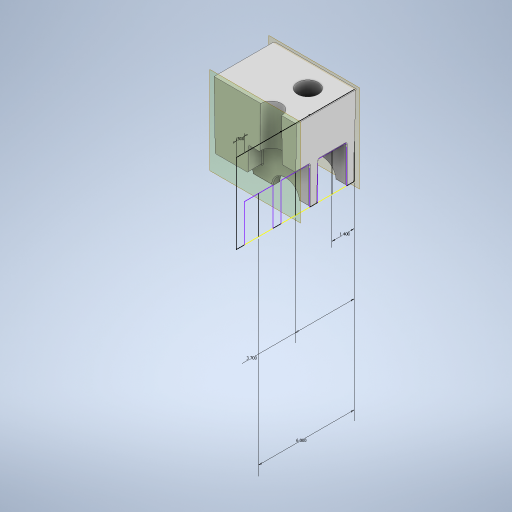
# Autodesk Inventor part: E.Engine Block Top Cast Image Left
Saved by Autodesk Inventor 2023 (Build 270158000, 158)
## iProperties
Created: 2023-01-04
Part Number: E.Engine Block Top Cast Image Left
Material: Generic
Document SubType Name: Modeling
Designer: tgr41
Density: 1 g/cm^3
Appearance: Default
Mass: 2134.37 g
Surface Area: 1668.76 cm^2
Volume: 2134.37 cm^3
Author: tgr41
Autodesk Inventor part; units mm, degrees
ref_plane "YZ Plane" through (0, 0, 0) normal (1, 0, 0) x (0, 1, 0)
ref_plane "XZ Plane" through (0, 0, 0) normal (0, 1, 0) x (-1, 0, 0)
sketch "Sketch1" plane through (0, 0, 0) normal (0, 0, 1) x (1, 0, 0)
  line L0 (127, 0) -> (127, 127)
  line L1 (127, 127) -> (0, 127)
  line L2 (0, 127) -> (0, 0)
  arc A0 (109.5375, 0) -> (68.2625, 0) centre (88.9, 0) ccw
  arc A1 (36.3964, 0) -> (14.4, 0) centre (25.3982, 0) ccw
  line L3 (14.4, 0) -> (0, 0)
  line L4 (127, 0) -> (109.5375, 0)
  line L5 (68.2625, 0) -> (36.3964, 0)
  dimension "d0" = 127
  dimension "d2" = 41.275
  dimension "d25" = 38.1
  dimension "d26" = 21.9964
  dimension "d30" = 127
  constraints: 12 end point, 4 point on circle, 3 horizontal, 2 centre point, 1 parallel
  measures "d0" distance of L1.end L0.end
  measures "d2" diameter of A0
  measures "d25" distance from line of L0 A0.centre
  measures "d26" diameter of A1
  measures "d30" distance between parallel lines of L1 L3
extrude "Extrusion1" add sketch "Sketch1" along normal blind 187.96
sketch "Sketch2" plane through (0, 127, 0) normal (0, 1, 0) x (1, 0, 0)
  circle A0 centre (88.9, -152.4) radius 17.78
  line L0 (127, -187.96) -> (0, -187.96) projected
  line L1 (127, 0) -> (127, -187.96) projected
  circle A1 centre (88.9, -93.98) radius 17.78
  circle A2 centre (88.9, -35.56) radius 17.78
  line L2 (127, 0) -> (0, 0) projected
  point P0 (127, -35.56)
  point P1 (127, -93.98)
  point P2 (127, -152.4)
  dimension "d6" = 35.56
  dimension "d7" = 38.1
  dimension "d10" = 35.56
  dimension "d11" = 38.1
  dimension "d13" = 58.42
  dimension "d14" = 38.1
  dimension "d29" = 35.56
  constraints: 3 centre point, 2 equal radius, 2 point on line, 1 midpoint
  measures "d6" distance from line of L0 A0.centre
  measures "d7" distance from line of L1 A0.centre
  measures "d10" distance from line of L2 A2.centre
  measures "d11" distance from line of L1 A2.centre
  measures "d13" distance of A1.centre A0.centre
  measures "d14" distance from line of L1 A1.centre
  measures "d29" diameter of A2
sketch "Sketch3" plane through (127, 0, 0) normal (1, 0, 0) x (0, 0, -1)
  line L0 (0, 127) -> (-187.96, 127) projected
  line L1 (0, 0) -> (-187.96, 0) projected
  line L2 (-35.56, 59.69) -> (-35.56, 0)
  line L3 (0, 0) -> (-187.96, 0) projected
  line L4 (-93.98, 0) -> (-93.98, 59.69)
  line L5 (-152.4, 59.69) -> (-152.4, 0)
  line L6 (0, 0) -> (0, 127) projected
  line L7 (-187.96, 0) -> (-175.26, 0)
  line L8 (-175.26, 0) -> (-175.26, 59.69)
  line L9 (-175.26, 127) -> (-187.96, 127)
  line L10 (-187.96, 127) -> (-187.96, 0)
  line L11 (-116.84, 0) -> (-129.54, 0)
  line L12 (-129.54, 0) -> (-129.54, 59.69)
  line L13 (-129.54, 127) -> (-116.84, 127)
  line L14 (-116.84, 59.69) -> (-116.84, 0)
  line L15 (-35.56, 59.69) -> (-35.56, 0)
  line L16 (0, 0) -> (-12.7, 0)
  line L17 (-12.7, 0) -> (-12.7, 59.69)
  line L18 (-12.7, 127) -> (0, 127)
  line L19 (0, 127) -> (0, 0)
  line L20 (-71.12, 0) -> (-58.42, 0)
  line L21 (-58.42, 0) -> (-58.42, 59.69)
  line L22 (-58.42, 127) -> (-71.12, 127)
  line L23 (-71.12, 59.69) -> (-71.12, 0)
  line L24 (-187.96, 127) -> (-187.96, 0) projected
  line L25 (-187.96, 127) -> (0, 127)
  line L26 (-58.42, 59.69) -> (-12.7, 59.69)
  line L27 (-175.26, 59.69) -> (-129.54, 59.69)
  line L28 (-116.84, 59.69) -> (-71.12, 59.69)
  dimension "d15" = 35.56
  dimension "d16" = 93.98
  dimension "d17" = 152.4
  dimension "d18" = 12.7
  constraints: 48 end point, 14 symmetric about line, 7 perpendicular, 4 midpoint, 3 point on line, 2 horizontal, 2 parallel
  measures "d15" distance between parallel lines of L6 L2
  measures "d16" distance between parallel lines of L6 L4
  measures "d17" distance between parallel lines of L6 L5
  measures "d18" distance of L9.end L9.start
extrude "Extrusion2" cut sketch "Sketch3" against normal blind 187.96 contours L1 L2 L26 L17 | L1 L21 L26 L2 | L1 L4 L28 L23 | L1 L14 L28 L4 | L1 L5 L27 L12 | L8 L27 L5 L1
extrude "Extrusion3" cut sketch "Sketch2" against normal blind 187.96
sketch "Sketch4" plane through (127, 59.69, 129.54) normal (0, -1, 0) x (1, 0, 0)
  line L0 (-58.7375, -116.84) -> (-90.6036, -116.84) projected
  line L1 (-74.6705, -116.84) -> (-74.6705, 45.72)
  line L2 (-90.6036, 45.72) -> (-58.7375, 45.72) projected
  line L3 (-74.6705, 45.72) -> (-127, 45.72)
  line L4 (-127, -116.84) -> (-127, -71.12) projected
  line L5 (-127, 45.72) -> (-127, -116.84)
  line L6 (-127, -116.84) -> (-74.6705, -116.84)
  point P0 (-127, -129.54)
  point P1 (-127, -71.12)
  constraints: 8 end point, 2 midpoint, 1 collinear, 1 horizontal, 1 perpendicular
extrude "Extrusion4" add sketch "Sketch4" along normal blind 38.1
draft "FaceDraft1" angle -1 pull direction (0, 1, 0) faces at (69.5273, 91.0988, 187.96) (0, 91.8633, 86.36) (127, 104.5633, 86.36) (69.5273, 91.0988, 0) (106.6223, 82.1267, 36.9907) (106.6223, 82.1267, 95.4107) (106.6223, 82.1267, 153.8307) fixed edges at (52.3295, 0, 187.96) (0, 0, 64.77) (127, 0, 6.35) (52.3295, 0, 0) (71.12, 59.69, 35.56) (71.12, 59.69, 93.98) (71.12, 59.69, 152.4)
draft "FaceDraft2" angle 1 pull direction (0, -1, 0) faces at (90.5863, 46.6223, 116.84) (90.5863, 46.6223, 129.54) fixed edges at (52.3295, 0, 116.84) (52.3295, 0, 129.54)
draft "FaceDraft3" angle 1 pull direction (0, -1, 0) faces at (90.5863, 46.6223, 58.42) (90.5863, 46.6223, 71.12) fixed edges at (118.2687, 0, 58.42) (118.2687, 0, 71.12)
draft "FaceDraft4" angle 1 pull direction (0, -1, 0) faces at (90.5863, 46.6223, 12.7) fixed edges at (52.3295, 0, 12.7)
draft "FaceDraft5" angle 1 pull direction (0, -1, 0) faces at (90.5863, 46.6223, 175.26) fixed edges at (52.3295, 0, 175.26)
draft "FaceDraft6" angle 1 pull direction (0, -1, 0) faces at (52.3295, 34.29, 42.8327) (52.3295, 34.29, 101.2527) (52.3295, 34.29, 159.6727) fixed edges at (52.3295, 21.59, 35.56) (52.3295, 21.59, 93.98) (52.3295, 21.59, 152.4)
fillet "Fillet1" radius 1.5875 89 edges at (52.9945, 59.69, 152.4) (52.662, 40.64, 130.2494) (90.5182, 59.69, 130.5819) (52.9945, 59.69, 93.98) (52.662, 40.64, 71.8294) (90.5182, 59.69, 72.1619) (90.5182, 59.69, 13.7419) (52.9945, 59.69, 35.56) (52.662, 40.64, 13.4094) (90.5182, 59.69, 174.2181) (52.662, 40.64, 174.5506) (90.5182, 59.69, 57.3781) (52.662, 40.64, 57.7106) (90.5182, 59.69, 115.7981) (52.662, 40.64, 116.1306) (25.9763, 21.59, 116.4631) (25.9763, 21.59, 174.8831) (25.9763, 21.59, 58.0431) (52.3295, 21.59, 35.56) (52.3295, 21.59, 93.98) (52.3295, 21.59, 152.4) (25.9763, 21.59, 129.9169) (25.9763, 21.59, 71.4969) (25.9763, 21.59, 13.0769) (71.12, 59.69, 35.56) (71.12, 59.69, 93.98) (71.12, 59.69, 152.4) (88.9, 20.6375, 129.9002) (118.2688, 0, 129.54) (118.2688, 0, 116.84) (88.9, 20.6375, 116.4798) (52.3295, 0, 116.84) (52.3295, 0, 129.54) (7.2, 0, 116.84) (7.2, 0, 129.54) (25.3982, 10.9982, 129.732) (25.3982, 10.9982, 116.648) (25.3982, 10.9982, 175.068) (7.2, 0, 175.26) (7.2, 0, 187.96) (25.3982, 10.9982, 188.152) (52.3295, 0, 175.26) (52.3295, 0, 187.96) (88.9, 20.6375, 174.8998) (88.9, 20.6375, 188.3202) (118.2688, 0, 187.96) (118.2687, 0, 175.26) (7.2, 0, 71.12) (25.3982, 10.9982, 71.312) (7.2, 0, 58.42) (25.3982, 10.9982, 58.228) (52.3295, 0, 58.42) (52.3295, 0, 71.12) (88.9, 20.6375, 58.0598) (88.9, 20.6375, 71.4802) (118.2687, 0, 71.12) (118.2688, 0, 58.42) (118.2687, 0, 12.7) (118.2688, 0, 0) (88.9, 20.6375, -0.3602) (88.9, 20.6375, 13.0602) (52.3295, 0, 0) (52.3295, 0, 12.7) (25.3982, 10.9982, -0.192) (25.3982, 10.9982, 12.892) (7.2, 0, 12.7) (7.2, 0, 0) (-0.3769, 21.59, 152.4) (-0.3769, 21.59, 93.98) (-0.3769, 21.59, 35.56) (128.0419, 59.69, 35.56) (128.0419, 59.69, 93.98) (128.0419, 59.69, 152.4) (-0.1884, 10.795, 58.2316) (-0.1884, 10.795, 71.3084) (-0.1884, 10.795, 116.6516) (-0.1884, 10.795, 175.0716) (-1.1084, 63.5, 189.0684) (-1.1084, 63.5, -1.1084) (-0.1884, 10.795, 12.8884) (128.1084, 63.5, -1.1084) (128.1084, 63.5, 189.0684) (127.5209, 29.845, 174.7391) (127.5209, 29.845, 130.0609) (127.5209, 29.845, 116.3191) (127.5209, 29.845, 71.6409) (127.5209, 29.845, 57.8991) (127.5209, 29.845, 13.2209) (-0.1884, 10.795, 129.7284)
ref_plane "Work Plane1" through (127.6295, -5384.1106, 93.98) normal (0, 0, -1) x (1, 0, 0)
sketch "Sketch5" plane through (127.6295, -5384.1106, 93.98) normal (0, 0, -1) x (1, 0, 0)
  line L0 (14.3742, -5369.3075) -> (-149.3252, -5369.3075)
  line L1 (-149.3252, -5369.3075) -> (-149.3252, -5529.1093)
  line L2 (-149.3252, -5529.1093) -> (14.3742, -5529.1093)
  line L3 (14.3742, -5529.1093) -> (14.3742, -5369.3075)
  point P0 (-127.6295, -5384.1106)
  constraints: 8 end point, 2 parallel, 1 horizontal, 1 perpendicular
extrude "Extrusion5" cut sketch "Sketch5" against normal blind 228.6
body "Solid1"
